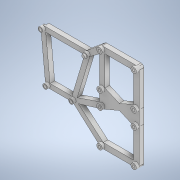
# Autodesk Inventor part: ElectronicsPlate
Saved by Autodesk Inventor 2021 (Build 250183000, 183)
## iProperties
Created: 2021-03-23
Part Number: ElectronicsPlate
Material: Generic
Document SubType Name: Modeling
Designer: elmar
Density: 1 g/cm^3
Appearance: Default
Author: elmar
Autodesk Inventor part; units mm, degrees
ref_plane "YZ Plane" through (0, 0, 0) normal (1, 0, 0) x (0, 1, 0)
ref_plane "XZ Plane" through (0, 0, 0) normal (0, 1, 0) x (-1, 0, 0)
ref_plane "XY Plane" through (0, 0, 0) normal (0, 0, 1) x (1, 0, 0)
sketch "Sketch1" plane through (0, 0, 0) normal (0, 0, 1) x (1, 0, 0)
  line L0 (26.67, -34.29) -> (-26.67, -34.29)
  line L1 (-26.67, -34.29) -> (-26.67, 34.29)
  line L2 (-26.67, 34.29) -> (26.67, 34.29)
  line L3 (26.67, 34.29) -> (26.67, -34.29)
  line L4 (26.67, -34.29) -> (-26.67, 34.29) construction
  line L5 (-26.67, -34.29) -> (26.67, 34.29) construction
  point P0 (0, 0)
  dimension "d0" = 68.58
  dimension "d1" = 53.34
  constraints: 12 end point, 2 midpoint, 2 parallel, 1 horizontal, 1 perpendicular
  measures "d0" distance of L0.end L1.end
  measures "d1" distance of L1.end L2.end
extrude "Extrusion1" add sketch "Sketch1" along normal blind 5
sketch "Sketch2" plane through (0, 0, 5) normal (0, 0, 1) x (1, 0, 0)
  line L0 (26.67, 34.29) -> (-26.67, 34.29) projected
  line L1 (-26.67, 34.29) -> (-26.67, -34.29) projected
  point P0 (0, 0)
  point P1 (-24.13, 19.05)
  point P2 (24.13, 19.05)
  point P3 (8.89, -31.75)
  point P4 (-19.05, -31.75)
  dimension "d4" = 15.24
  dimension "d5" = 15.24
  dimension "d6" = 2.54
  dimension "d7" = 50.8
  dimension "d8" = 7.62
  dimension "d9" = 66.04
  dimension "d10" = 66.04
  dimension "d11" = 35.56
  measures "d4" distance from line of L0 point (-24.13, 19.05)
  measures "d5" distance from line of L0 point (24.13, 19.05)
  measures "d6" distance from line of point (-24.13, 19.05) L1
  measures "d7" distance from line of L1 point (24.13, 19.05)
  measures "d8" distance from line of point (-19.05, -31.75) L1
  measures "d9" distance from line of point (-19.05, -31.75) L0
  measures "d10" distance from line of L0 point (8.89, -31.75)
  measures "d11" distance from line of point (8.89, -31.75) L1
hole "Hole1" at (-24.13, 19.05, 5) at (24.13, 19.05, 5) at (8.89, -31.75, 5) at (-19.05, -31.75, 5) direction (0, 0, -1) diameter 3.2 end through all clearance for "Flat Head Machine Screw" size "M3" standard "Ansi Metric M Profile"
sketch "Sketch3" plane through (0, 0, 5) normal (0, 0, 1) x (1, 0, 0)
  circle A0 centre (-24.13, 19.05) radius 1.6 projected
  circle A1 centre (24.13, 19.05) radius 1.6 projected
  circle A2 centre (-19.05, -31.75) radius 1.6 projected
  circle A3 centre (8.89, -31.75) radius 1.6 projected
  circle A4 centre (-24.13, 19.05) radius 2.54
  circle A5 centre (24.13, 19.05) radius 2.54
  circle A6 centre (-19.05, -31.75) radius 2.54
  circle A7 centre (8.89, -31.75) radius 2.54
  line L0 (-26.67, 34.29) -> (-26.67, -34.29) projected
  line L1 (-26.67, -34.29) -> (26.67, -34.29) projected
  line L2 (26.67, -34.29) -> (26.67, 34.29) projected
  point P0 (0, 0)
  constraints: 4 centre point, 4 coincident, 4 tangent
extrude "Extrusion2" add sketch "Sketch3" along normal blind 3
sketch "Sketch4" plane through (0, 0, 0) normal (0, 0, -1) x (-1, 0, 0)
  circle A0 centre (-8.89, -31.75) radius 1.6 projected
  circle A1 centre (19.05, -31.75) radius 1.6 projected
  circle A2 centre (24.13, 19.05) radius 1.6 projected
  line L0 (21.38, 17.4623) -> (21.38, 20.6377)
  line L1 (21.38, 20.6377) -> (24.13, 22.2254)
  line L2 (24.13, 22.2254) -> (26.88, 20.6377)
  line L3 (26.88, 20.6377) -> (26.88, 17.4623)
  line L4 (26.88, 17.4623) -> (24.13, 15.8746)
  line L5 (24.13, 15.8746) -> (21.38, 17.4623)
  line L6 (17.4623, -29) -> (20.6377, -29)
  line L7 (20.6377, -29) -> (22.2254, -31.75)
  line L8 (22.2254, -31.75) -> (20.6377, -34.5)
  line L9 (20.6377, -34.5) -> (17.4623, -34.5)
  line L10 (17.4623, -34.5) -> (15.8746, -31.75)
  line L11 (15.8746, -31.75) -> (17.4623, -29)
  line L12 (-10.4777, -29) -> (-7.3023, -29)
  line L13 (-7.3023, -29) -> (-5.7146, -31.75)
  line L14 (-5.7146, -31.75) -> (-7.3023, -34.5)
  line L15 (-7.3023, -34.5) -> (-10.4777, -34.5)
  line L16 (-10.4777, -34.5) -> (-12.0654, -31.75)
  line L17 (-12.0654, -31.75) -> (-10.4777, -29)
  point P0 (0, 0)
  dimension "d23" = 5.5
  constraints: 36 end point, 3 coincident, 2 horizontal, 2 perpendicular, 1 vertical, 39 other
  measures "d23" distance between parallel lines of L3 L0
extrude "Extrusion3" cut sketch "Sketch4" against normal blind 3 contours A2 | L0 L1 L2 L3 L4 L5 | L6 L7 L8 L9 L10 L11 | L12 L13 L14 L15 L16 L17
sketch "Sketch5" plane through (0, 0, 0) normal (0, 0, -1) x (-1, 0, 0)
  circle A0 centre (-24.13, 19.05) radius 1.6 projected
  point P0 (0, 0)
extrude "Extrusion4" add sketch "Sketch5" against normal blind 10
sketch "Sketch6" plane through (0, 0, 0) normal (0, 0, 1) x (1, 0, 0)
  line L0 (26.67, -34.29) -> (26.67, 34.29) projected
  line L1 (26.67, 34.29) -> (79.67, 34.29)
  line L2 (79.67, 34.29) -> (79.67, -61.71)
  line L3 (79.67, -61.71) -> (26.67, -61.71)
  line L4 (26.67, -61.71) -> (26.67, 34.29)
  point P0 (0, 0)
  dimension "d28" = 53
  dimension "d29" = 96
  constraints: 8 end point, 2 parallel, 1 horizontal, 1 perpendicular
  measures "d28" distance of L0.end L1.end
  measures "d29" distance of L1.end L2.end
extrude "Extrusion5" add sketch "Sketch6" along normal up to surface (5 mm away)
sketch "Sketch7" plane through (0, 0, 5) normal (0, 0, 1) x (1, 0, 0)
  line L0 (76.67, 31.29) -> (39.67, 31.29)
  line L1 (39.67, 31.29) -> (39.67, -5.71)
  line L2 (39.67, -5.71) -> (76.67, -5.71)
  line L3 (76.67, -5.71) -> (76.67, 31.29)
  line L4 (79.67, 34.29) -> (79.67, -61.71) projected
  line L5 (-26.67, 34.29) -> (79.67, 34.29) projected
  point P0 (0, 0)
  dimension "d32" = 37
  dimension "d33" = 3
  dimension "d34" = 3
  constraints: 8 end point, 2 parallel, 2 perpendicular, 1 horizontal
  measures "d32" distance of L0.end L1.end
  measures "d33" distance between parallel lines of L4 L3
  measures "d34" distance between parallel lines of L0 L5
hole "Hole2" at (76.67, 31.29, 5) direction (0, 0, -1) diameter 2.7 end through all clearance for "Flat Head Machine Screw" size "M2.5" standard "Ansi Metric M Profile"
sketch "Sketch8" plane through (0, 0, 5) normal (0, 0, 1) x (1, 0, 0)
  circle A0 centre (76.67, 31.29) radius 1.35 projected
  circle A1 centre (76.67, 31.29) radius 3
  line L0 (79.67, 34.29) -> (-26.67, 34.29) projected
  point P0 (0, 0)
  constraints: 1 centre point, 1 coincident, 1 tangent
extrude "Extrusion6" add sketch "Sketch8" along normal blind 3
sketch "Sketch9" plane through (0, 0, 0) normal (0, 0, -1) x (-1, 0, 0)
  circle A0 centre (-76.67, 31.29) radius 1.35 projected
  line L0 (-78.1134, 33.79) -> (-75.2266, 33.79)
  line L1 (-75.2266, 33.79) -> (-73.7832, 31.29)
  line L2 (-73.7832, 31.29) -> (-75.2266, 28.79)
  line L3 (-75.2266, 28.79) -> (-78.1134, 28.79)
  line L4 (-78.1134, 28.79) -> (-79.5568, 31.29)
  line L5 (-79.5568, 31.29) -> (-78.1134, 33.79)
  point P0 (0, 0)
  dimension "d44" = 5
  constraints: 12 end point, 1 coincident, 1 horizontal, 13 other
  measures "d44" distance between parallel lines of L2 L5
extrude "Extrusion7" cut sketch "Sketch9" against normal blind 3
pattern_linear "Rectangular Pattern1" count 2 spacing 37 along (-1, 0, 0) count 2 spacing 37 along (0, -1, 0) of "Extrusion6", "Extrusion7", "Hole2"
pattern_linear "Rectangular Pattern2" count 2 spacing 53 along (0, -1, 0) of "Extrusion6", "Extrusion7", "Hole2", "Rectangular Pattern1"
sketch "Sketch10" plane through (0, 0, 5) normal (0, 0, 1) x (1, 0, 0)
  arc A0 (79.67, -58.71) -> (76.67, -61.71) centre (76.67, -58.71) ccw projected
  line L0 (79.67, -21.71) -> (79.67, -58.71) projected
  circle A1 centre (76.67, -21.71) radius 3 projected
  line L1 (79.67, -5.71) -> (79.67, -21.71) projected
  circle A2 centre (76.67, -5.71) radius 3 projected
  line L2 (79.67, 31.29) -> (79.67, -5.71) projected
  arc A3 (76.67, 34.29) -> (79.67, 31.29) centre (76.67, 31.29) ccw projected
  line L3 (39.67, 34.29) -> (76.67, 34.29) projected
  circle A4 centre (39.67, 31.29) radius 3 projected
  line L4 (-26.67, 34.29) -> (39.67, 34.29) projected
  line L5 (-26.67, 34.29) -> (-26.67, 19.05) projected
  circle A5 centre (-24.13, 19.05) radius 2.54 projected
  line L6 (-26.67, 19.05) -> (-26.67, -34.29) projected
  line L7 (-26.67, -34.29) -> (-19.05, -34.29) projected
  circle A6 centre (-19.05, -31.75) radius 2.54 projected
  line L8 (-19.05, -34.29) -> (8.89, -34.29) projected
  circle A7 centre (8.89, -31.75) radius 2.54 projected
  line L9 (8.89, -34.29) -> (26.67, -34.29) projected
  line L10 (26.67, -61.71) -> (26.67, -34.29) projected
  line L11 (39.67, -61.71) -> (26.67, -61.71) projected
  circle A8 centre (39.67, -58.71) radius 3 projected
  circle A9 centre (24.13, 19.05) radius 2.54 projected
  circle A10 centre (39.67, -5.71) radius 3 projected
  circle A11 centre (39.67, -21.71) radius 3 projected
  line L12 (-24.13, 21.59) -> (24.13, 21.59)
  circle A12 centre (24.13, 19.05) radius 2.54 projected
  line L13 (37.7594, 33.6029) -> (22.5124, 21.0083)
  circle A13 centre (39.67, 31.29) radius 3 projected
  circle A14 centre (-24.13, 19.05) radius 2.54 projected
  line L14 (-21.6026, 19.3027) -> (-16.5226, -31.4973)
  line L15 (-21.5774, -32.0027) -> (-26.6574, 18.7973)
  circle A15 centre (-19.05, -31.75) radius 2.54 projected
  circle A16 centre (-19.05, -31.75) radius 2.54 projected
  line L16 (-19.05, -29.21) -> (8.89, -29.21)
  line L17 (8.0681, -29.3467) -> (38.6993, -18.8714)
  circle A17 centre (39.67, -21.71) radius 3 projected
  circle A18 centre (39.67, -58.71) radius 3 projected
  line L18 (39.67, -55.71) -> (76.67, -55.71)
  arc A19 (79.67, -58.71) -> (76.67, -61.71) centre (76.67, -58.71) ccw projected
  line L19 (73.67, -58.71) -> (73.67, 31.29)
  line L20 (39.67, 28.29) -> (76.67, 28.29)
  circle A20 centre (39.67, 31.29) radius 3 projected
  line L21 (42.67, 31.29) -> (42.67, -58.71)
  circle A21 centre (8.89, -31.75) radius 2.54 projected
  circle A22 centre (39.67, -21.71) radius 3 projected
  line L22 (9.6433, -34.1757) -> (40.5597, -24.575)
  line L23 (-24.13, 16.51) -> (24.13, 16.51)
  line L24 (25.6548, 17.0186) -> (41.471, 28.8907)
  line L25 (36.67, 31.29) -> (36.67, -58.71)
  circle A23 centre (39.67, -5.71) radius 3 projected
  circle A24 centre (76.67, -21.71) radius 3 projected
  circle A25 centre (76.67, -5.71) radius 3 projected
  line L26 (38.4793, -8.4636) -> (75.4793, -24.4636)
  circle A26 centre (24.13, 19.05) radius 2.54 projected
  circle A27 centre (39.67, -58.71) radius 3 projected
  circle A28 centre (76.67, -58.71) radius 3 projected
  line L27 (21.6971, 19.7799) -> (6.4571, -31.0201)
  circle A29 centre (8.89, -31.75) radius 2.54 projected
  line L28 (11.3229, -32.4799) -> (26.5629, 18.3201)
  line L29 (7.1951, -33.6418) -> (37.6681, -60.9444)
  line L30 (76.67, 34.29) -> (79.67, 34.29) projected
  line L31 (79.67, 34.29) -> (79.67, 31.29) projected
  line L32 (79.67, -61.71) -> (76.67, -61.71) projected
  line L33 (79.67, -58.71) -> (79.67, -61.71) projected
  line L34 (79.67, -58.71) -> (79.67, -61.71) projected
  line L35 (76.67, -61.71) -> (39.67, -61.71) projected
  arc A30 (76.67, -61.71) -> (79.67, -58.71) centre (76.67, -58.71) ccw projected
  line L36 (79.67, -61.71) -> (76.67, -61.71) projected
  line L37 (10.542, -29.8206) -> (41.6212, -56.4312)
  line L38 (40.8607, -24.4636) -> (77.8607, -8.4636)
  line L39 (40.8607, -2.9564) -> (77.8607, -18.9564)
  line L40 (38.4793, -18.9564) -> (75.4793, -2.9564)
  point P0 (0, 0)
  point P1 (37.6681, -60.9444)
  point P2 (26.67, -46.0238)
  point P3 (36.67, -18.8682)
  point P4 (73.67, -23.6812)
  point P5 (42.67, -55.71)
  point P6 (73.67, -55.71)
  point P7 (73.67, 28.29)
  point P8 (42.67, 28.29)
  point P9 (26.3229, 17.5201)
  point P10 (12.7424, -27.7481)
  point P11 (36.67, -19.5654)
  point P12 (36.67, 25.287)
  point P13 (7.0002, -29.21)
  point P14 (20.7162, 16.51)
  point P15 (-21.3233, 16.51)
  point P16 (-16.7513, -29.21)
  point P17 (-26.6574, 18.7973)
  point P18 (23.2166, 21.59)
  point P19 (8.153, -34.29)
  point P20 (36.67, -25.7829)
  point P21 (42.67, -10.2758)
  point P22 (26.67, -51.0905)
  point P23 (7.9186, -34.29)
  point P24 (58.17, -10.4415)
  point P25 (73.67, -3.7388)
  point P26 (42.67, -3.7388)
  point P27 (58.17, -16.9785)
  point P28 (42.67, -23.6812)
  point P29 (14.0355, -32.8118)
  point P30 (15.7619, -34.29)
  point P31 (26.67, -43.6297)
  point P32 (40.7789, -55.71)
  point P33 (36.67, -25.7829)
  point P34 (36.67, -52.1919)
  constraints: 44 end point, 41 tangent, 37 point on circle, 4 point on line, 2 horizontal, 2 perpendicular, 1 horizontal alignment, 1 parallel, 16 other
extrude "Extrusion8" cut sketch "Sketch10" against normal through all contours L18 L21 L38 L26 L19 | L11 L10 L29 A8 | L18 L37 L25 L22 A11 L38 L21 | L40 L39 L21 L20 L19 | L37 L10 L9 L22 L25 | L37 L9 L10 | A4 L13 L12 A5 L5 L4 | L7 L6 A5 L15 A6 | L17 L28 L24 L25 | L16 L14 L23 L27
fillet "Fillet1" radius 3 2 edges at (79.67, 34.29, 2.5) (79.67, -61.71, 2.5)
extrude "Extrusion9" add sketch "Sketch10" against normal up to surface (5 mm away) contours L29 L8 L9 L37 L10
body "Solid1"
